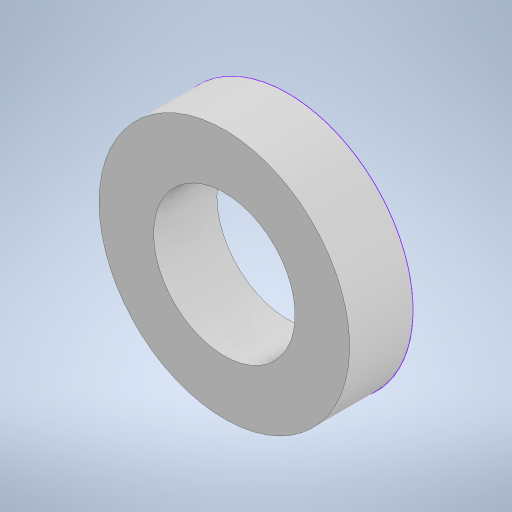
# Autodesk Inventor part: test part
Saved by Autodesk Inventor 2024 (Build 280153000, 153)
## iProperties
Created: 2024-09-19
Part Number: test part
Material: Generic
Document SubType Name: Modeling
Designer: thatg
Density: 1 g/cm^3
Appearance: Default
Author: thatg
Autodesk Inventor part; units mm, degrees
ref_plane "YZ Plane" through (0, 0, 0) normal (1, 0, 0) x (0, 1, 0)
ref_plane "XZ Plane" through (0, 0, 0) normal (0, 1, 0) x (-1, 0, 0)
ref_plane "XY Plane" through (0, 0, 0) normal (0, 0, 1) x (1, 0, 0)
sketch "Sketch1" plane through (0, 0, 0) normal (0, 1, 0) x (-1, 0, 0)
  line L0 (0, 0) -> (13.518, 0)
  line L1 (13.518, 0) -> (13.518, -15.5818)
  line L2 (13.518, -15.5818) -> (0, -15.5818)
  line L3 (0, -15.5818) -> (0, 0)
  line L4 (13.1878, 0) -> (7.4504, 0)
  line L5 (7.4504, 0) -> (7.4504, -6.6661)
  line L6 (7.4504, -6.6661) -> (13.1878, -6.6661)
  line L7 (13.1878, -6.6661) -> (13.1878, 0)
  line L8 (6.3359, -10.4223) -> (3.0338, -10.4223)
  line L9 (3.0338, -10.4223) -> (3.0338, -12.8163)
  line L10 (3.0338, -12.8163) -> (6.3359, -12.8163)
  line L11 (6.3359, -12.8163) -> (6.3359, -10.4223)
  constraints: 24 end point, 6 parallel, 3 horizontal, 3 perpendicular, 1 point on line
revolve "Revolution1" add sketch "Sketch1" angle 360 about axis through (0, 0, -15.5818) along (0, 0, 1) contours L0 L7 L6 L5
sketch "Sketch2" plane through (0, 0, -6.6661) normal (0, 0, -1) x (-1, 0, 0)
  circle A0 centre (0, 0) radius 13.1878
  constraints: 1 centre point, 1 coincident
body "Solid1"
